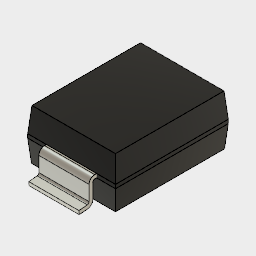
TSOP-2+4mm (Autodesk Fusion 360 design; units mm, degrees)
Autodesk Fusion 360 part; units mm, degrees
ref_plane "WorkPlane1" through (0, 0, 0.925) normal (0, 0, 1) x (1, 0, 0)
sketch "Sketch1" plane through (0, 0, 0.925) normal (0, 0, 1) x (1, 0, 0)
  line L0 (1.75, 2.25) -> (-1.75, 2.25)
  line L1 (-1.75, 2.25) -> (-1.75, -2.25)
  line L2 (-1.75, -2.25) -> (1.75, -2.25)
  line L3 (1.75, -2.25) -> (1.75, 2.25)
  line L4 (1.75, 2.25) -> (-1.75, -2.25) construction
  line L5 (-1.75, 2.25) -> (1.75, -2.25) construction
  dimension "d2" = 3.5
  dimension "d3" = 4.5
  measures "d2" distance of L1.end L2.end
  measures "d3" distance of L0.end L1.end
extrude "Extrude1" add sketch "Sketch1" against normal blind 0.875 draft -5 makes body 1
extrude "Extrude3" add sketch "Sketch1" along normal blind 0.15 bodies 1
extrude "Extrude4" add sketch "Sketch1" along normal blind 0.975 draft -5 from surface at 0.15 bodies 1
sketch "Sketch2" plane through (0, -2.25, 0) normal (0, -1, 0) x (1, 0, 0)
  line L0 (1.4672, 0.1123) -> (1.5, 0.4887)
  line L1 (1, 0.925) -> (-1, 0.925)
  line L2 (-1, 0.925) -> (-1, 1.075)
  line L3 (-1, 1.075) -> (1, 1.075)
  line L4 (1, 1.075) -> (1, 0.925)
  line L5 (1, 0.925) -> (-1, 1.075) construction
  line L6 (-1, 0.925) -> (1, 1.075) construction
  line L7 (-1.75, 0.925) -> (1.75, 0.925)
  line L8 (1.75, 0.925) -> (1.75, 1.075)
  line L9 (1.75, 1.075) -> (-1.75, 1.075)
  line L10 (-1.75, 1.075) -> (-1.75, 0.925)
  point P0 (0, 1)
  dimension "d6" = 2
  dimension "d7" = 0.15
  dimension "d51" = 1
  measures "d6" distance of L2.end L3.end
  measures "d7" distance of L1.end L2.end
  measures "d51" distance of origin P0
sketch "Sketch3" plane through (0, 0, 0) normal (1, 0, 0) x (0, 1, 0)
  line L0 (-2.25, 1) -> (-2.325, 1)
  arc A0 (-2.325, 1) -> (-2.475, 0.85) centre (-2.325, 0.85) ccw
  line L1 (-2.475, 0.85) -> (-2.475, 0.254)
  arc A1 (-2.6119, 0.1046) -> (-2.475, 0.254) centre (-2.625, 0.254) ccw
  line L2 (-2.6119, 0.1046) -> (-2.95, 0.075)
  line L3 (-2.25, 1.075) -> (-2.25, 0.925)
  line L4 (-2.25, 1) -> (-2.1, 1)
  line L5 (-2.95, 0.075) -> (-2.45, 0.075) construction
  point P0 (-2.25, 1)
  dimension "d10" = 0.15
  dimension "d11" = 0.075
  dimension "d21" = 0.15
  dimension "d22" = 0.225
  dimension "d23" = 0.7
  dimension "d24" = 0.5
  dimension "d25" = 5
  dimension "d26" = 0.15
  measures "d10" radius of A0
  measures "d11" distance of origin L2.end
  measures "d21" distance of P0 L4.end
  measures "d22" distance of P0 L1
  measures "d23" distance of P0 L2.end
  measures "d24" distance of L2.end L5.end
  measures "d25" angle of L2 L5
  measures "d26" radius of A1
sweep "Sweep1" add profiles "Sketch2" path "Sketch3" along L2 A1 L1 A0 L0 L4 section 1 contours L1 L2 L3 L4 L7 L9 separate body makes body 2
mirror "Mirror1" about plane through (0, 0, 0) normal (0, 1, 0) of "Sweep1" makes body 3
equation "d1 = tsop2_4_lead_attach - tsop2_4_lead_thickness / 2"
equation "d2 = tsop2_4_package_width"
equation "d3 = tsop2_4_package_depth"
equation "d4 = -tsop2_4_lead_attach + tsop2_4_lead_thickness / 2 + tsop2_4_above_board"
equation "d5 = -tsop2_4_package_taper"
equation "d6 = tsop2_4_lead_width"
equation "d7 = tsop2_4_lead_thickness"
equation "d10 = tsop2_4_lead_thickness"
equation "d11 = tsop2_4_lead_thickness / 2"
equation "tsop2_4_lead_thickness = 0.15 mm"
equation "tsop2_4_lead_attach = 1 mm"
equation "tsop2_4_lead_width = 2 mm"
equation "tsop2_4_lead_spacing = 1 mm"
equation "tsop2_4_package_width = 3.5 mm"
equation "tsop2_4_package_height = 2 mm"
equation "tsop2_4_package_depth = 4.5 mm"
equation "tsop2_4_above_board = 0.05 mm"
equation "d21 = tsop2_4_lead_into_package"
equation "d22 = tsop2_4_lead_thickness * ( 3 / 2 )"
equation "d23 = tsop2_4_lead_extension"
equation "d25 = tsop2_4_lead_foot_angle"
equation "d26 = d10"
equation "tsop2_4_lead_extension = 0.7 mm"
equation "tsop2_4_lead_foot_angle = 5 deg"
equation "tsop2_4_lead_into_package = 0.15 mm"
equation "tsop2_4_optional_lead_extension = 0 mm"
equation "tsop2_4_package_taper = 5 deg"
equation "d46 = tsop2_4_lead_thickness"
equation "d48 = tsop2_4_lead_thickness"
equation "d49 = tsop2_4_package_height - tsop2_4_lead_thickness / 2 - ( tsop2_4_lead_attach - tsop2_4_above_board )"
equation "d50 = -tsop2_4_package_taper"
equation "d51 = tsop2_4_lead_attach"
named bodies: "lead2", "opt_lead"
